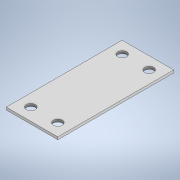
# Autodesk Inventor part: adaptdor cnc
Saved by Autodesk Inventor 2021 (Build 250183000, 183)
## iProperties
Created: 2022-10-08
Part Number: adaptdor cnc
Material: Genérico
Document SubType Name: Modeling
Designer: sergi
Density: 1 g/cm^3
Appearance: Valor por defecto
Author: sergi
Autodesk Inventor part; units mm, degrees
ref_plane "YZ Plane" through (0, 0, 0) normal (1, 0, 0) x (0, 1, 0)
ref_plane "XZ Plane" through (0, 0, 0) normal (0, 1, 0) x (-1, 0, 0)
ref_plane "XY Plane" through (0, 0, 0) normal (0, 0, 1) x (1, 0, 0)
sketch "Boceto1" plane through (0, 0, 0) normal (0, 1, 0) x (-1, 0, 0)
  line L0 (-20, -45) -> (20, -45)
  line L1 (20, -45) -> (20, 45)
  line L2 (20, 45) -> (-20, 45)
  line L3 (-20, 45) -> (-20, -45)
  line L4 (-20, -45) -> (20, 45) construction
  line L5 (20, -45) -> (-20, 45) construction
  point P0 (0, 0)
  dimension "d0" = 40
  dimension "d1" = 90
  constraints: 12 end point, 2 midpoint, 2 parallel, 1 horizontal, 1 perpendicular
  measures "d0" distance of L2.end L1.end
  measures "d1" distance of L1.end L0.end
extrude "Extrusión1" add sketch "Boceto1" along normal blind 2
sketch "Boceto2" plane through (0, 2, 0) normal (0, 1, 0) x (1, 0, 0)
  line L0 (-20, 45) -> (-20, -45) projected
  line L1 (-20, -45) -> (20, -45) projected
  line L2 (20, -45) -> (20, 45) projected
  line L3 (20, 45) -> (-20, 45) projected
  point P0 (0, 0)
  point P1 (-10.5, -35.5)
  point P2 (10.5, -35.5)
  point P3 (-10.5, 35.5)
  point P4 (10.5, 35.5)
  dimension "d4" = 9.5
  dimension "d5" = 9.5
  dimension "d6" = 9.5
  dimension "d7" = 9.5
  dimension "d8" = 9.5
  dimension "d9" = 9.5
  dimension "d10" = 9.5
  dimension "d11" = 9.5
  measures "d4" distance from line of L0 point (-10.5, -35.5)
  measures "d5" distance from line of L1 point (-10.5, -35.5)
  measures "d6" distance from line of L2 point (10.5, -35.5)
  measures "d7" distance from line of L1 point (10.5, -35.5)
  measures "d8" distance from line of L3 point (-10.5, 35.5)
  measures "d9" distance from line of L0 point (-10.5, 35.5)
  measures "d10" distance from line of L3 point (10.5, 35.5)
  measures "d11" distance from line of L2 point (10.5, 35.5)
hole "Agujero1" at (-10.5, 2, 35.5) at (10.5, 2, 35.5) at (-10.5, 2, -35.5) at (10.5, 2, -35.5) direction (0, -1, 0) diameter 7 end through all
